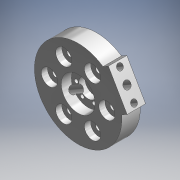
# Autodesk Inventor part: AA046
Saved by Autodesk Inventor 2017 SP1 (Build 210196100, 196)
## iProperties
Created: 2018-01-29
Part Number: AA046
Material: ABS Plastic
Document SubType Name: Modeling
Designer: Zach
Density: 1.06 g/cm^3
Appearance: CR White
Author: Zach
Autodesk Inventor part; units mm, degrees
ref_plane "YZ Plane" through (0, 0, 0) normal (1, 0, 0) x (0, 1, 0)
ref_plane "XZ Plane" through (0, 0, 0) normal (0, 1, 0) x (-1, 0, 0)
ref_plane "XY Plane" through (0, 0, 0) normal (0, 0, 1) x (1, 0, 0)
sketch "Sketch1" plane through (0, 0, 0) normal (0, 0, 1) x (1, 0, 0)
  circle A0 centre (0, 0) radius 35
  circle A1 centre (0, 0) radius 4.5
  dimension "d0" = 70
  dimension "d1" = 9
  constraints: 2 centre point, 2 coincident
  measures "d0" diameter of A0
  measures "d1" diameter of A1
extrude "Extrusion1" add sketch "Sketch1" along normal blind 14.75
sketch "Sketch2" plane through (0, 0, 14.75) normal (0, 0, 1) x (1, 0, 0)
  circle A0 centre (0, 0) radius 13.5
  dimension "d4" = 27
  constraints: 1 centre point, 1 coincident
  measures "d4" diameter of A0
extrude "Extrusion2" cut sketch "Sketch2" against normal blind 8
sketch "Sketch3" plane through (0, 0, 6.75) normal (0, 0, 1) x (1, 0, 0)
  circle A0 centre (0, 0) radius 7.5
  dimension "d7" = 15
  constraints: 1 centre point, 1 coincident
  measures "d7" diameter of A0
extrude "Extrusion3" cut sketch "Sketch3" against normal blind 5
sketch "Sketch4" plane through (0, 0, 6.75) normal (0, 0, 1) x (1, 0, 0)
  circle A0 centre (9.525, 0) radius 1.5
  circle A1 centre (4.7625, 8.2489) radius 1.5
  circle A2 centre (-4.7625, 8.2489) radius 1.5
  circle A3 centre (-9.525, 0) radius 1.5
  circle A4 centre (-4.7625, -8.2489) radius 1.5
  circle A5 centre (4.7625, -8.2489) radius 1.5
  point P0 (0, 0)
  dimension "d10" = 3
  dimension "d11" = 9.525
  dimension "d14" = 360
  constraints: 6 centre point, 1 horizontal alignment, 13 other
  measures "d10" diameter of A0
  measures "d11" distance of A0.centre point (0, 0)
extrude "Extrusion4" cut sketch "Sketch4" against normal through all
sketch "Sketch5" plane through (0, 0, 14.75) normal (0, 0, 1) x (1, 0, 0)
  circle A0 centre (23, 0) radius 2.5
  circle A1 centre (11.5, 19.9186) radius 2.5
  circle A2 centre (-11.5, 19.9186) radius 2.5
  circle A3 centre (-23, 0) radius 2.5
  circle A4 centre (-11.5, -19.9186) radius 2.5
  circle A5 centre (11.5, -19.9186) radius 2.5
  point P0 (0, 0)
  dimension "d18" = 5
  dimension "d19" = 23
  dimension "d22" = 360
  constraints: 6 centre point, 1 horizontal alignment, 13 other
  measures "d18" diameter of A0
  measures "d19" distance of A0.centre point (0, 0)
extrude "Extrusion5" cut sketch "Sketch5" against normal through all
sketch "Sketch6" plane through (0, 0, 14.75) normal (0, 0, 1) x (1, 0, 0)
  circle A0 centre (23, 0) radius 2.5 projected
  circle A1 centre (23, 0) radius 6.5
  circle A2 centre (11.5, 19.9186) radius 6.5
  circle A3 centre (-11.5, 19.9186) radius 6.5
  circle A4 centre (-23, 0) radius 6.5
  circle A5 centre (-11.5, -19.9186) radius 6.5
  circle A6 centre (11.5, -19.9186) radius 6.5
  point P0 (0, 0)
  dimension "d26" = 13
  dimension "d29" = 360
  constraints: 6 centre point, 1 coincident, 13 other
  measures "d26" diameter of A1
extrude "Extrusion6" cut sketch "Sketch6" against normal blind 5 contours A0 | A1 | A2 | A3 | A4 | A5 | A6
sketch "Sketch7" plane through (0, 0, 14.75) normal (0, 0, 1) x (1, 0, 0)
  line L0 (19.8861, 28.8018) -> (24.2163, 31.3018)
  line L1 (24.2163, 31.3018) -> (39.2163, 5.321)
  line L2 (39.2163, 5.321) -> (34.8861, 2.821)
  line L3 (34.8861, 2.821) -> (19.8861, 28.8018)
  circle A0 centre (0, 0) radius 35 construction
  line L4 (0, 0) -> (27.3861, 15.8114)
  circle A1 centre (23, 0) radius 2.5 construction
  line L5 (0, 0) -> (23, 0)
  dimension "d33" = 5
  dimension "d34" = 30
  dimension "d43" = 30
  constraints: 12 end point, 2 parallel, 2 point on circle, 1 horizontal, 1 midpoint, 1 perpendicular
  measures "d33" distance of L0.start L0.end
  measures "d34" distance of L0.end L1.end
  measures "d43" angle of L5 L4
extrude "Extrusion7" add sketch "Sketch7" against normal blind 14.75
sketch "Sketch8" plane through (39.2163, 5.321, 14.75) normal (0.8660254, 0.5, 0) x (0, 0, -1)
  circle A0 centre (7.375, 26.25) radius 2.5
  circle A1 centre (7.375, 3.75) radius 2.5
  line L0 (7.375, 26.25) -> (7.375, 3.75) construction
  line L1 (14.75, 30) -> (14.75, 0) projected
  line L2 (0, 30) -> (14.75, 30) projected
  point P0 (14.75, 15)
  point P1 (14.75, 15)
  point P2 (7.375, 15)
  point P3 (7.375, 30)
  dimension "d37" = 5
  dimension "d38" = 5
  dimension "d39" = 22.5
  constraints: 3 midpoint, 2 centre point, 2 end point, 1 horizontal alignment, 1 vertical, 1 vertical alignment
  measures "d37" diameter of A0
  measures "d38" diameter of A1
  measures "d39" distance of L0.start L0.end
extrude "Extrusion8" cut sketch "Sketch8" against normal blind 10
sketch "Sketch9" plane through (39.2163, 5.321, 14.75) normal (0.8660254, 0.5, 0) x (0, 0, -1)
  circle A0 centre (7.375, 15) radius 3
  line L0 (14.75, 30) -> (14.75, 0) projected
  circle A1 centre (7.375, 26.25) radius 2.5 construction
  point P0 (14.75, 15)
  point P1 (14.75, 15)
  dimension "d42" = 6
  constraints: 1 centre point, 1 horizontal alignment, 1 midpoint, 1 vertical alignment
  measures "d42" diameter of A0
extrude "Extrusion9" cut sketch "Sketch9" against normal through all
body "Solid1"
